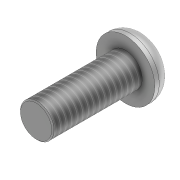
# Autodesk Inventor part: Tornillo Allen cabeza botón M6x16mm
Saved by Autodesk Inventor 2020.3 (Build 243373000, 373)
## iProperties
Created: 2020-05-16
Part Number: Tornillo Allen cabeza botón M6x16mm
Material: Generic
Document SubType Name: Modeling
Designer: Dante
Density: 1 g/cm^3
Appearance: Rubber - Black - Version 1.1
Mass: 0.788426 g
Surface Area: 6.87968 cm^2
Volume: 0.788426 cm^3
Author: Dante
Autodesk Inventor part; units mm, degrees
ref_plane "YZ Plane" through (0, 0, 0) normal (1, 0, 0) x (0, 1, 0)
ref_plane "XZ Plane" through (0, 0, 0) normal (0, 1, 0) x (-1, 0, 0)
ref_plane "XY Plane" through (0, 0, 0) normal (0, 0, 1) x (1, 0, 0)
sketch "Sketch1" plane through (0, 0, 0) normal (0, 0, 1) x (1, 0, 0)
  circle A0 centre (0, 0) radius 3
  circle A1 centre (0, 0) radius 5.25
  dimension "d0" = 6
  dimension "d1" = 10.5
  constraints: 2 centre point, 2 coincident
  measures "d0" diameter of A0
  measures "d1" diameter of A1
extrude "Extrusion1" add sketch "Sketch1" along normal blind 0.8
extrude "Extrusion2" add sketch "Sketch1" along normal blind 16.8 contours A0
thread "Thread1" size "M6x1" class "6g" standard "ANSI Metric M Profile" length 348
sketch "Boceto3" plane through (0, 0, 0) normal (0, 0, -1) x (-1, 0, 0)
  circle A0 centre (0, 0) radius 5.25
  constraints: 1 centre point, 1 coincident
extrude "Extrusión3" add sketch "Boceto3" along normal blind 2.5
fillet "Empalme2" radius 2.5 1 edges at (5.25, 0, -2.5)
sketch "Boceto4" plane through (0, 0, -2.5) normal (0, 0, -1) x (-1, 0, 0)
  line L0 (-2.2122, -1.978) -> (-2.8191, 0.9269)
  line L1 (-2.8191, 0.9269) -> (-0.6069, 2.9049)
  line L2 (-0.6069, 2.9049) -> (2.2122, 1.978)
  line L3 (2.2122, 1.978) -> (2.8191, -0.9269)
  line L4 (2.8191, -0.9269) -> (0.6069, -2.9049)
  line L5 (0.6069, -2.9049) -> (-2.2122, -1.978)
  point P0 (0, 0)
  point P1 (0, 0)
  dimension "d12" = 5.14
  constraints: 12 end point, 1 coincident, 13 other
  measures "d12" distance between parallel lines of L1 L4
extrude "Extrusión4" cut sketch "Boceto4" against normal blind 2.5
chamfer "Chaflán1" distance 0.2 angle 45 1 edges at (-3, 0, 16.8)
body "Solid1"
